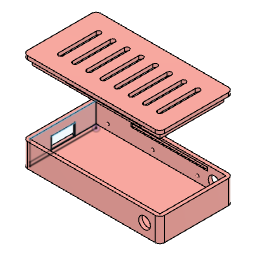
Case 003 v6 (Autodesk Fusion 360 design; units mm, degrees)
Autodesk Fusion 360 part; units mm, degrees
sketch "Bodemplaat" plane through (0, 0, 0) normal (0, 1, 0) x (1, 0, 0)
  line L0 (0, 0) -> (55, 0)
  line L1 (55, 0) -> (55, -28)
  line L2 (55, -28) -> (0, -28)
  line L3 (0, -28) -> (0, 0)
  line L4 (54.5, -29.5) -> (0.5, -29.5)
  line L5 (-1.5, -27.5) -> (-1.5, -0.5)
  line L6 (0.5, 1.5) -> (54.5, 1.5)
  line L7 (56.5, -0.5) -> (56.5, -27.5)
  arc A0 (0.5, 1.5) -> (-1.5, -0.5) centre (0.5, -0.5) ccw
  arc A1 (-1.5, -27.5) -> (0.5, -29.5) centre (0.5, -27.5) ccw
  arc A2 (54.5, -29.5) -> (56.5, -27.5) centre (54.5, -27.5) ccw
  arc A3 (56.5, -0.5) -> (54.5, 1.5) centre (54.5, -0.5) ccw
  dimension "d1" = 55
  dimension "d2" = 28
  dimension "d4" = 2
  constraint horizontal L0
  constraint vertical L1
  constraint horizontal L2
  constraint vertical L3
  constraint coincident L0.start L3.end
  constraint parallel L2 L4
  constraint parallel L3 L5
  constraint parallel L0 L6
  constraint parallel L1 L7
  constraint tangent L5 A0
  constraint tangent L6 A0
  constraint tangent L4 A1
  constraint tangent L5 A1
  constraint equal A0 A1
  constraint tangent L4 A2
  constraint tangent L7 A2
  constraint equal A0 A2
  constraint tangent L6 A3
  constraint tangent L7 A3
  constraint equal A0 A3
  measures "d1" distance of L0.start L0.end
  measures "d2" distance of L0.start L2.end
  measures "d4" radius of A0
sketch "Deksel" plane through (0, 0, 0) normal (0, 1, 0) x (-1, 0, 0)
  line L0 (0, 0) -> (-55, 0)
  line L1 (-55, 0) -> (-55, 28)
  line L2 (-55, 28) -> (0, 28)
  line L3 (0, 28) -> (0, 0)
  line L4 (-54.5, 29.5) -> (-0.5, 29.5)
  line L5 (1.5, 27.5) -> (1.5, 0.5)
  line L6 (-0.5, -1.5) -> (-54.5, -1.5)
  line L7 (-56.5, 0.5) -> (-56.5, 27.5)
  arc A0 (-0.5, -1.5) -> (1.5, 0.5) centre (-0.5, 0.5) ccw
  arc A1 (1.5, 27.5) -> (-0.5, 29.5) centre (-0.5, 27.5) ccw
  arc A2 (-54.5, 29.5) -> (-56.5, 27.5) centre (-54.5, 27.5) ccw
  arc A3 (-56.5, 0.5) -> (-54.5, -1.5) centre (-54.5, 0.5) ccw
  line L8 (-54.5, 27.5) -> (-0.5, 27.5)
  line L9 (-0.5, 27.5) -> (-0.5, 0.5)
  line L10 (-0.5, 0.5) -> (-54.5, 0.5)
  line L11 (-54.5, 0.5) -> (-54.5, 27.5)
  line L12 (-53, 26) -> (-2, 26)
  line L13 (-2, 26) -> (-2, 2)
  line L14 (-2, 2) -> (-53, 2)
  line L15 (-53, 2) -> (-53, 26)
  line L16 (0, 14) -> (-55, 14)
  line L17 (-6.0117, 6) -> (-6.0117, 22)
  arc A4 (-6.0117, 22) -> (-8.0117, 22) centre (-7.0117, 22) ccw
  line L18 (-8.0117, 22) -> (-8.0117, 6)
  arc A5 (-8.0117, 6) -> (-6.0117, 6) centre (-7.0117, 6) ccw
  line L19 (-7.0117, 6) -> (-7.0117, 22) construction
  line L20 (-13.0117, 6) -> (-13.0117, 22) construction
  arc A6 (-14.0117, 6) -> (-12.0117, 6) centre (-13.0117, 6) ccw
  line L21 (-14.0117, 22) -> (-14.0117, 6)
  arc A7 (-12.0117, 22) -> (-14.0117, 22) centre (-13.0117, 22) ccw
  line L22 (-12.0117, 6) -> (-12.0117, 22)
  line L23 (-19.0117, 6) -> (-19.0117, 22) construction
  line L24 (-25.0117, 6) -> (-25.0117, 22) construction
  line L25 (-20.0117, 22) -> (-20.0117, 6)
  line L26 (-18.0117, 6) -> (-18.0117, 22)
  arc A8 (-24.0117, 22) -> (-26.0117, 22) centre (-25.0117, 22) ccw
  line L27 (-26.0117, 22) -> (-26.0117, 6)
  arc A9 (-20.0117, 6) -> (-18.0117, 6) centre (-19.0117, 6) ccw
  line L28 (-24.0117, 6) -> (-24.0117, 22)
  arc A10 (-18.0117, 22) -> (-20.0117, 22) centre (-19.0117, 22) ccw
  arc A11 (-26.0117, 6) -> (-24.0117, 6) centre (-25.0117, 6) ccw
  line L29 (-49.0117, 6) -> (-49.0117, 22) construction
  line L30 (-50.0117, 22) -> (-50.0117, 6)
  line L31 (-48.0117, 6) -> (-48.0117, 22)
  arc A12 (-48.0117, 22) -> (-50.0117, 22) centre (-49.0117, 22) ccw
  arc A13 (-50.0117, 6) -> (-48.0117, 6) centre (-49.0117, 6) ccw
  line L32 (-37.0117, 6) -> (-37.0117, 22) construction
  line L33 (-30.0117, 6) -> (-30.0117, 22)
  arc A14 (-30.0117, 22) -> (-32.0117, 22) centre (-31.0117, 22) ccw
  arc A15 (-36.0117, 22) -> (-38.0117, 22) centre (-37.0117, 22) ccw
  arc A16 (-32.0117, 6) -> (-30.0117, 6) centre (-31.0117, 6) ccw
  arc A17 (-38.0117, 6) -> (-36.0117, 6) centre (-37.0117, 6) ccw
  line L34 (-32.0117, 22) -> (-32.0117, 6)
  line L35 (-38.0117, 22) -> (-38.0117, 6)
  line L36 (-31.0117, 6) -> (-31.0117, 22) construction
  line L37 (-36.0117, 6) -> (-36.0117, 22)
  line L38 (-44.0117, 22) -> (-44.0117, 6)
  arc A18 (-42.0117, 22) -> (-44.0117, 22) centre (-43.0117, 22) ccw
  line L39 (-42.0117, 6) -> (-42.0117, 22)
  arc A19 (-44.0117, 6) -> (-42.0117, 6) centre (-43.0117, 6) ccw
  line L40 (-43.0117, 6) -> (-43.0117, 22) construction
  point P0 (-7.0117, 14)
  point P1 (-13.0117, 14)
  point P2 (-25.0117, 14)
  point P3 (-19.0117, 14)
  point P4 (-49.0117, 14)
  point P5 (-43.0117, 14)
  point P6 (-37.0117, 14)
  point P7 (-31.0117, 14)
  dimension "d5" = 55
  dimension "d6" = 28
  dimension "d8" = 2
  dimension "d9" = 0.5
  dimension "d18" = 2
  dimension "d40" = 2
  dimension "d41" = 2
  dimension "d42" = 2
  dimension "d43" = 2
  dimension "d44" = 2
  dimension "d45" = 2
  dimension "d46" = 2
  dimension "d47" = 2
  constraint horizontal L0
  constraint vertical L1
  constraint horizontal L2
  constraint vertical L3
  constraint coincident L0.start L3.end
  constraint parallel L2 L4
  constraint parallel L3 L5
  constraint parallel L0 L6
  constraint parallel L1 L7
  constraint tangent L5 A0
  constraint tangent L6 A0
  constraint tangent L4 A1
  constraint tangent L5 A1
  constraint equal A0 A1
  constraint tangent L4 A2
  constraint tangent L7 A2
  constraint equal A0 A2
  constraint tangent L6 A3
  constraint tangent L7 A3
  constraint equal A0 A3
  constraint midpoint L3 L16.start
  constraint midpoint L1 L16.end
  constraint tangent L17 A4
  constraint tangent A4 L18
  constraint parallel L17 L18
  constraint tangent L18 A5
  constraint tangent L17 A5
  constraint perpendicular L16 L19
  constraint coincident L16 P0
  constraint midpoint L19 P0
  constraint tangent A7 L22
  constraint tangent L21 A7
  constraint parallel L21 L22
  constraint tangent A6 L21
  constraint tangent A6 L22
  constraint midpoint P1 L20
  constraint tangent L26 A10
  constraint tangent L25 A10
  constraint parallel L25 L26
  constraint tangent L25 A9
  constraint tangent L26 A9
  constraint midpoint P3 L23
  constraint tangent A8 L28
  constraint tangent A8 L27
  constraint parallel L27 L28
  constraint tangent L27 A11
  constraint tangent L28 A11
  constraint midpoint P2 L24
  constraint tangent L33 A14
  constraint tangent A14 L34
  constraint parallel L33 L34
  constraint tangent A16 L34
  constraint tangent L33 A16
  constraint midpoint P7 L36
  constraint tangent A15 L37
  constraint tangent A15 L35
  constraint parallel L35 L37
  constraint tangent A17 L35
  constraint tangent A17 L37
  constraint midpoint P6 L32
  constraint tangent A18 L39
  constraint tangent L38 A18
  constraint parallel L38 L39
  constraint tangent L38 A19
  constraint tangent L39 A19
  constraint midpoint P5 L40
  constraint tangent L31 A12
  constraint tangent L30 A12
  constraint parallel L30 L31
  constraint tangent L30 A13
  constraint tangent L31 A13
  constraint midpoint P4 L29
  measures "d5" distance of L0.start L0.end
  measures "d6" distance of L0.start L2.end
  measures "d8" radius of A0
  measures "d40" diameter of A4
  measures "d41" diameter of A7
  measures "d42" diameter of A10
  measures "d43" diameter of A8
  measures "d44" diameter of A14
  measures "d45" diameter of A15
  measures "d46" diameter of A18
  measures "d47" diameter of A12
extrude "Extrude1" add sketch "Bodemplaat" along normal blind 1.5 contours L0 L1 L2 L3 makes body 1
extrude "Extrude2" add sketch "Bodemplaat" along normal blind 10 bodies 1
ref_plane "WorkPlane1" through (27.5, 40, 14) normal (0, 1, 0) x (-1, 0, 0)
extrude "Extrude3" add sketch "Deksel" along normal blind 1.5 from surface at 40 separate body contours L0 L1 L3 L9 L10 L11 L16 | L1 L2 L3 L8 L9 L11 L16 | L8 L9 L11 L12 L13 L15 L16 | L9 L10 L11 L13 L14 L15 L16 | L12 L13 L15 L16 L17 A4 L18 L21 A7 L22 L25 L26 A8 L27 L28 A10 L30 L31 A12 L33 A14 A15 L34 L35 L37 L38 A18 L39 | L13 L14 L15 L16 L17 L18 A5 A6 L21 L22 L25 L26 L27 A9 L28 A11 L30 L31 A13 L33 A16 A17 L34 L35 L37 L38 L39 A19 | L16 L17 L18 A5 | L16 L17 A4 L18 | L16 L30 L31 A12 | L16 L30 L31 A13 | L16 A6 L21 L22 | L16 L21 A7 L22 | L16 L38 A18 L39 | L16 L38 L39 A19 | L16 L25 L26 A9 | L16 L25 L26 A10 | L16 A15 L35 L37 | L16 A17 L35 L37 | L16 L27 L28 A11 | L16 A8 L27 L28 | L16 L33 A14 L34 | L16 L33 A16 L34 | L4 L5 L6 L7 A0 A1 A2 A3 makes body 2
extrude "Extrude4" add sketch "Deksel" against normal blind 3 from surface at 40 contours L8 L9 L11 L12 L13 L15 L16 | L9 L10 L11 L13 L14 L15 L16 bodies 2
sketch "Zijkant" plane through (0, 0, 0) normal (0, 0, 1) x (1, 0, 0)
  line L0 (0, 0) -> (55, 0)
  line L1 (55, 0) -> (55, 10)
  line L2 (55, 10) -> (0, 10)
  line L3 (0, 10) -> (0, 0)
  line L4 (0, 40) -> (55, 40)
  line L5 (55, 40) -> (55, 37)
  line L6 (55, 37) -> (0, 37)
  line L7 (0, 37) -> (0, 40)
  line L8 (15, 9) -> (47, 9)
  line L9 (47, 9) -> (47, 8)
  line L10 (47, 8) -> (15, 8)
  line L11 (15, 8) -> (15, 9)
  line L12 (15, 39) -> (47, 39)
  line L13 (47, 39) -> (47, 38)
  line L14 (47, 38) -> (15, 38)
  line L15 (15, 38) -> (15, 39)
  line L16 (47.2, 7.8) -> (14.8, 7.8)
  line L17 (14.8, 7.8) -> (14.8, 9.2)
  line L18 (14.8, 9.2) -> (47.2, 9.2)
  line L19 (47.2, 9.2) -> (47.2, 7.8)
  dimension "d29" = -0.2
  constraint horizontal L0
  constraint vertical L1
  constraint horizontal L2
  constraint vertical L3
  constraint coincident L0.start L3.end
  constraint horizontal L4
  constraint vertical L5
  constraint horizontal L6
  constraint vertical L7
  constraint horizontal L8
  constraint vertical L9
  constraint horizontal L10
  constraint vertical L11
  constraint horizontal L12
  constraint vertical L13
  constraint horizontal L14
  constraint vertical L15
extrude "Extrude7" cut sketch "Zijkant" against normal blind 0.5 contours L8 L9 L10 L11 | L16 L17 L18 L19 bodies 1
extrude "Extrude8" cut sketch "Zijkant" along normal blind 0.5 from surface at 28 contours L8 L9 L10 L11 | L16 L17 L18 L19 bodies 1
extrude "Extrude6" add sketch "Zijkant" against normal blind 0.75 from surface at 0.5 contours L12 L13 L14 L15 bodies 2
extrude "Extrude9" add sketch "Zijkant" along normal blind 0.75 from surface at 27.5 contours L12 L13 L14 L15 bodies 2
fillet "Fillet1" radius 0.5 8 edges at (31, 39, -0.25) (31, 38, -0.25) (15, 38.5, -0.25) (47, 38.5, -0.25) (31, 39, 28.25) (15, 38.5, 28.25) (31, 38, 28.25) (47, 38.5, 28.25) on bodies 2
extrude "Extrude10" cut sketch "Deksel" against normal up to surface (1.5 mm away) from surface at 41.5 contours L16 L17 L18 A5 | L16 L17 A4 L18 | L16 L30 L31 A12 | L16 L30 L31 A13 | L16 A6 L21 L22 | L16 L21 A7 L22 | L16 L38 A18 L39 | L16 L38 L39 A19 | L16 L25 L26 A9 | L16 L25 L26 A10 | L16 A15 L35 L37 | L16 A17 L35 L37 | L16 L27 L28 A11 | L16 A8 L27 L28 | L16 L33 A14 L34 | L16 L33 A16 L34 bodies 2
cylinder "CylinderPrimitive2" cut diameter 5 height -31 placed x (1, 0, 0) y (0, 1, 0) z (0, 0, 1) at (50, 5, 29.5) bodies 1
sketch "Sketch6" plane through (0, 0, 0) normal (1, 0, 0) x (0, 0, -1)
  line L0 (0, 0) -> (-28, 0)
  line L1 (-28, 0) -> (-28, 10)
  line L2 (-28, 10) -> (0, 10)
  line L3 (0, 10) -> (0, 0)
  line L4 (0, 0) -> (-28, 0)
  line L5 (-28, 0) -> (-28, 1.5)
  line L6 (-28, 1.5) -> (0, 1.5)
  line L7 (0, 1.5) -> (0, 0)
  line L8 (-9, 6.5) -> (-19, 6.5)
  line L9 (-19, 6.5) -> (-19, 1.5)
  line L10 (-19, 1.5) -> (-9, 1.5)
  line L11 (-9, 1.5) -> (-9, 6.5)
  dimension "d55" = 28
  dimension "d56" = 1.5
  dimension "d72" = 10
  dimension "d73" = 28
  constraint horizontal L0
  constraint vertical L1
  constraint horizontal L2
  constraint vertical L3
  constraint coincident L0.start L3.end
  constraint horizontal L4
  constraint vertical L5
  constraint horizontal L6
  constraint vertical L7
  constraint horizontal L8
  constraint vertical L9
  constraint horizontal L10
  constraint vertical L11
  constraint midpoint L6 L10
  measures "d55" distance of L0.start L0.end
  measures "d56" distance of L0.start L6.end
  measures "d72" distance of L8.start L8.end
  measures "d73" distance of L5.end L6.end
extrude "Extrude11" cut sketch "Sketch6" against normal up to surface (1.5 mm away) contours L6 L8 L9 L10 L11 bodies 1
fillet "Fillet2" radius 1 3 edges at (-1.5, 4, 9) (-1.5, 6.5, 14) (-1.5, 4, 19) on bodies 1
ref_plane "WorkPlane2" through (0, 4.5, 0) normal (0, 1, 0) x (0, 0, 1)
sphere "SpherePrimitive2" add diameter 1.15 placed x (1, 0, 0) y (0, 1, 0) z (0, 0, 1) at (5, 4, 0) bodies 1
pattern_linear "R-Pattern2" count 2 spacing 28 along (0, 0, 1) count 3 spacing 19 along (1, 0, 0) of "SpherePrimitive2"
named bodies: "Kast", "Deksel"
